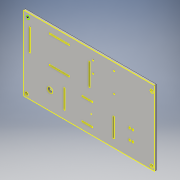
# Autodesk Inventor part: bottom
Saved by Autodesk Inventor 2016 (Build 200138000, 138)
## iProperties
Created: 2017-09-18
Part Number: bottom
Material: Generic
Document SubType Name: Modeling
Designer: Student
Density: 1 g/cm^3
Appearance: Default
Author: Student
Autodesk Inventor part; units mm, degrees
ref_plane "YZ Plane" through (0, 0, 0) normal (1, 0, 0) x (0, 1, 0)
ref_plane "XZ Plane" through (0, 0, 0) normal (0, 1, 0) x (-1, 0, 0)
ref_plane "XY Plane" through (0, 0, 0) normal (0, 0, 1) x (1, 0, 0)
sketch "Sketch1" plane through (0, 0, 0) normal (0, 0, 1) x (1, 0, 0)
  line L0 (-164.322, 128.7031) -> (152.924, 128.7031)
  line L1 (152.924, 128.7031) -> (152.924, -133.4523)
  line L2 (152.924, -133.4523) -> (-164.322, -133.4523)
  line L3 (-164.322, -133.4523) -> (-164.322, 128.7031)
  point P0 (0, 0)
  dimension "d0" = 317.246
  constraints: 8 end point, 2 parallel, 1 horizontal, 1 perpendicular
  measures "d0" distance of L0.start L0.end
extrude "Extrusion1" add sketch "Sketch1" along normal blind 4.699
sketch "Sketch2" plane through (0, 0, 4.699) normal (0, 0, 1) x (1, 0, 0)
  line L0 (-22.7697, 25.1619) -> (2.6303, 25.1619)
  line L1 (52.3147, 22.4498) -> (52.3147, -24.5402)
  line L2 (-64.5253, -24.5402) -> (-64.5253, 22.4498)
  line L3 (52.3147, 22.4498) -> (54.8547, 22.4498)
  line L4 (54.8547, 22.4498) -> (54.8547, -24.5402)
  line L5 (54.8547, -24.5402) -> (52.3147, -24.5402)
  line L6 (52.3147, -24.5402) -> (52.3147, 22.4498)
  line L7 (-64.5253, -24.5402) -> (-67.0653, -24.5402)
  line L8 (-67.0653, -24.5402) -> (-67.0653, 22.4498)
  line L9 (-67.0653, 22.4498) -> (-64.5253, 22.4498)
  line L10 (-64.5253, 22.4498) -> (-64.5253, -24.5402)
  line L11 (-22.7697, 25.1619) -> (2.6303, 25.1619)
  line L12 (2.6303, 25.1619) -> (2.6303, 27.7019)
  line L13 (2.6303, 27.7019) -> (-22.7697, 27.7019)
  line L14 (-22.7697, 27.7019) -> (-22.7697, 25.1619)
  line L15 (-22.7697, -25.2309) -> (2.6303, -25.2309)
  line L16 (2.6303, -25.2309) -> (2.6303, -27.7709)
  line L17 (2.6303, -27.7709) -> (-22.7697, -27.7709)
  line L18 (-22.7697, -27.7709) -> (-22.7697, -25.2309)
  circle A0 centre (92.5652, 17.0242) radius 2.286
  circle A1 centre (100.1852, 17.0242) radius 2.286
  circle A2 centre (92.5652, -8.3758) radius 2.286
  circle A3 centre (100.1852, -8.3758) radius 2.286
  line L19 (3.9163, 100.2262) -> (59.1645, 100.2262)
  circle A4 centre (54.7163, 69.5732) radius 1.397
  circle A5 centre (54.7163, 117.8332) radius 1.397
  circle A6 centre (3.9163, 114.6403) radius 1.397
  circle A7 centre (3.9163, 86.7003) radius 1.397
  point P0 (0, 0)
  dimension "d3" = 116.84
  dimension "d4" = 46.99
  dimension "d5" = 2.54
  dimension "d6" = 2.54
  dimension "d7" = 25.4
  dimension "d8" = 2.54
  dimension "d9" = 2.54
  dimension "d12" = 4.572
  dimension "d31" = 25.4
  dimension "d32" = 25.4
  constraints: 40 end point, 9 parallel, 8 centre point, 6 horizontal, 5 perpendicular, 1 point on line
  measures "d3" distance of L2.end L1.start
  measures "d4" distance of L1.start L1.end
  measures "d5" distance of L4.end L5.end
  measures "d6" distance of L8.end L9.end
  measures "d7" distance of L13.end L12.end
  measures "d8" distance of L0.end L12.end
  measures "d9" distance of L15.end L16.end
  measures "d12" diameter of A0
  measures "d31" distance of A3.centre A1.centre
  measures "d32" distance of A2.centre A0.centre
extrude "Extrusion2" cut sketch "Sketch2" against normal blind 25.4
sketch "Sketch3" plane through (0, 0, 4.699) normal (0, 0, 1) x (1, 0, 0)
  line L0 (-164.322, 128.7031) -> (-164.322, -133.4523) projected
  line L1 (152.924, 128.7031) -> (152.924, -133.4523) projected
  line L2 (-164.322, -44.2248) -> (152.924, -44.2248)
  line L3 (152.924, -44.2248) -> (152.924, -133.4523)
  line L4 (152.924, -133.4523) -> (-164.322, -133.4523)
  line L5 (-164.322, -133.4523) -> (-164.322, -44.2248)
  point P0 (0, 0)
  constraints: 8 end point, 2 parallel, 1 horizontal, 1 perpendicular, 1 point on line
extrude "Extrusion3" cut sketch "Sketch3" against normal blind 25.4
sketch "Sketch4" plane through (0, 0, 4.699) normal (0, 0, 1) x (1, 0, 0)
  line L0 (-102.2349, 116.84) -> (-53.5128, 116.84)
  line L1 (-6.2523, 108.1454) -> (-6.2523, 44.8408)
  line L2 (-53.5128, 53.5354) -> (-102.2349, 53.5354)
  line L3 (-148.4923, 53.5354) -> (-148.4923, 108.1454)
  line L4 (-148.4923, 108.1454) -> (-151.0323, 108.1454)
  line L5 (-151.0323, 108.1454) -> (-151.0323, 53.5354)
  line L6 (-151.0323, 53.5354) -> (-148.4923, 53.5354)
  line L7 (-148.4923, 53.5354) -> (-148.4923, 108.1454)
  line L8 (-6.2523, 108.1454) -> (-3.7123, 108.1454)
  line L9 (-3.7123, 108.1454) -> (-3.7123, 53.5354)
  line L10 (-3.7123, 53.5354) -> (-6.2523, 53.5354)
  line L11 (-6.2523, 53.5354) -> (-6.2523, 108.1454)
  line L12 (-102.2349, 116.84) -> (-53.5128, 116.84)
  line L13 (-53.5128, 116.84) -> (-53.5128, 119.5161)
  line L14 (-53.5128, 119.5161) -> (-102.2349, 119.5161)
  line L15 (-102.2349, 119.5161) -> (-102.2349, 116.84)
  line L16 (-102.2349, 53.5354) -> (-53.5128, 53.5354)
  line L17 (-53.5128, 53.5354) -> (-53.5128, 50.5868)
  line L18 (-53.5128, 50.5868) -> (-102.2349, 50.5868)
  line L19 (-102.2349, 50.5868) -> (-102.2349, 53.5354)
  circle A0 centre (-100.2931, 0) radius 6.35
  point P0 (0, 0)
  dimension "d21" = 142.24
  dimension "d22" = 2.54
  dimension "d23" = 2.54
  dimension "d24" = 12.7
  dimension "d25" = 54.61
  constraints: 40 end point, 10 parallel, 5 horizontal, 5 perpendicular, 3 point on line, 1 centre point
  measures "d21" distance of L3.end L1.start
  measures "d22" distance of L6.end L5.end
  measures "d23" distance of L9.end L10.end
  measures "d24" diameter of A0
  measures "d25" distance of L4.end L5.end
extrude "Extrusion4" cut sketch "Sketch4" against normal blind 25.4
sketch "Sketch5" plane through (0, 0, 4.699) normal (0, 0, 1) x (1, 0, 0)
  circle A0 centre (-154.2096, 125.6742) radius 4.064
  line L0 (-6.2523, 53.5354) -> (-6.2523, 108.1454) projected
  line L1 (-6.2523, 108.1454) -> (-3.7123, 108.1454) projected
  line L2 (-3.7123, 108.1454) -> (-3.7123, 53.5354) projected
  line L3 (-3.7123, 53.5354) -> (-6.2523, 53.5354) projected
  line L4 (-102.2349, 116.84) -> (-102.2349, 119.5161) projected
  line L5 (-102.2349, 119.5161) -> (-53.5128, 119.5161) projected
  line L6 (-53.5128, 119.5161) -> (-53.5128, 116.84) projected
  line L7 (-53.5128, 116.84) -> (-102.2349, 116.84) projected
  circle A1 centre (-100.2931, 0) radius 6.35 projected
  line L8 (-151.0323, 53.5354) -> (-151.0323, 108.1454) projected
  line L9 (-151.0323, 108.1454) -> (-148.4923, 108.1454) projected
  line L10 (-148.4923, 108.1454) -> (-148.4923, 53.5354) projected
  line L11 (-148.4923, 53.5354) -> (-151.0323, 53.5354) projected
  line L12 (-102.2349, 53.5354) -> (-53.5128, 53.5354) projected
  line L13 (-53.5128, 53.5354) -> (-53.5128, 50.5868) projected
  line L14 (-53.5128, 50.5868) -> (-102.2349, 50.5868) projected
  line L15 (-102.2349, 50.5868) -> (-102.2349, 53.5354) projected
  line L16 (-164.322, -44.2248) -> (152.924, -44.2248) projected
  line L17 (152.924, -44.2248) -> (152.924, 128.7031) projected
  line L18 (152.924, 128.7031) -> (-164.322, 128.7031) projected
  line L19 (-164.322, 128.7031) -> (-164.322, -44.2248) projected
  line L20 (-164.322, 128.7031) -> (152.924, 128.7031) projected
  line L21 (-5.699, 128.7031) -> (-5.699, 116.84)
  circle A2 centre (145.9955, 120.8351) radius 4.064
  line L22 (-164.322, -44.2248) -> (-164.322, 128.7031) projected
  line L23 (-164.322, 42.2392) -> (-157.3936, 42.2392)
  circle A3 centre (-157.3936, -36.3568) radius 4.064
  circle A4 centre (145.9955, -36.3568) radius 4.064
  point P0 (0, 0)
  dimension "d28" = 8.128
  constraints: 4 centre point, 4 end point, 2 midpoint, 1 horizontal, 1 symmetric about line, 1 vertical, 1 other
  measures "d28" diameter of A0
extrude "Extrusion5" cut sketch "Sketch5" against normal blind 25.4 contours A0 L18 | L18 A0 | A2 | A3 | A4
sketch "Sketch6" plane through (0, 0, 4.699) normal (0, 0, 1) x (1, 0, 0)
  circle A0 centre (-157.3936, -36.3568) radius 4.064 projected
  arc A1 (-156.9191, 128.7031) -> (-151.5, 128.7031) centre (-154.2096, 125.6742) ccw projected
  circle A2 centre (145.9955, 120.8351) radius 4.064 projected
  circle A3 centre (145.9955, -36.3568) radius 4.064 projected
  line L0 (-6.2523, 53.5354) -> (-6.2523, 108.1454) projected
  line L1 (-6.2523, 108.1454) -> (-3.7123, 108.1454) projected
  line L2 (-3.7123, 108.1454) -> (-3.7123, 53.5354) projected
  line L3 (-3.7123, 53.5354) -> (-6.2523, 53.5354) projected
  line L4 (-102.2349, 116.84) -> (-102.2349, 119.5161) projected
  line L5 (-102.2349, 119.5161) -> (-53.5128, 119.5161) projected
  line L6 (-53.5128, 119.5161) -> (-53.5128, 116.84) projected
  line L7 (-53.5128, 116.84) -> (-102.2349, 116.84) projected
  circle A4 centre (-100.2931, 0) radius 6.35 projected
  line L8 (-151.0323, 53.5354) -> (-151.0323, 108.1454) projected
  line L9 (-151.0323, 108.1454) -> (-148.4923, 108.1454) projected
  line L10 (-148.4923, 108.1454) -> (-148.4923, 53.5354) projected
  line L11 (-148.4923, 53.5354) -> (-151.0323, 53.5354) projected
  line L12 (-102.2349, 53.5354) -> (-53.5128, 53.5354) projected
  line L13 (-53.5128, 53.5354) -> (-53.5128, 50.5868) projected
  line L14 (-53.5128, 50.5868) -> (-102.2349, 50.5868) projected
  line L15 (-102.2349, 50.5868) -> (-102.2349, 53.5354) projected
  line L16 (-164.322, -44.2248) -> (152.924, -44.2248) projected
  line L17 (152.924, -44.2248) -> (152.924, 128.7031) projected
  line L18 (152.924, 128.7031) -> (-151.5, 128.7031) projected
  line L19 (-164.322, 128.7031) -> (-164.322, -44.2248) projected
  line L20 (-64.5253, 22.4498) -> (-64.5253, -24.5402) projected
  line L21 (-64.5253, -24.5402) -> (-67.0653, -24.5402) projected
  line L22 (-67.0653, -24.5402) -> (-67.0653, 22.4498) projected
  line L23 (-67.0653, 22.4498) -> (-64.5253, 22.4498) projected
  line L24 (-22.7697, -27.7709) -> (-22.7697, -25.2309) projected
  line L25 (-22.7697, -25.2309) -> (2.6303, -25.2309) projected
  line L26 (2.6303, -25.2309) -> (2.6303, -27.7709) projected
  line L27 (2.6303, -27.7709) -> (-22.7697, -27.7709) projected
  circle A5 centre (100.1852, -8.3758) radius 2.286 projected
  circle A6 centre (100.1852, 17.0242) radius 2.286 projected
  circle A7 centre (54.7163, 117.8332) radius 1.397 projected
  circle A8 centre (54.7163, 69.5732) radius 1.397 projected
  circle A9 centre (3.9163, 86.7003) radius 1.397 projected
  circle A10 centre (3.9163, 114.6403) radius 1.397 projected
  circle A11 centre (92.5652, 17.0242) radius 2.286 projected
  circle A12 centre (92.5652, -8.3758) radius 2.286 projected
  line L28 (-22.7697, 25.1619) -> (-22.7697, 27.7019) projected
  line L29 (-22.7697, 27.7019) -> (2.6303, 27.7019) projected
  line L30 (2.6303, 27.7019) -> (2.6303, 25.1619) projected
  line L31 (2.6303, 25.1619) -> (-22.7697, 25.1619) projected
  line L32 (52.3147, -24.5402) -> (52.3147, 22.4498) projected
  line L33 (52.3147, 22.4498) -> (54.8547, 22.4498) projected
  line L34 (54.8547, 22.4498) -> (54.8547, -24.5402) projected
  line L35 (54.8547, -24.5402) -> (52.3147, -24.5402) projected
  line L36 (-164.322, 128.7031) -> (152.924, 128.7031) projected
  line L37 (-164.322, 128.7031) -> (152.924, 128.7031)
  line L38 (152.924, 128.7031) -> (152.924, 136.3029)
  line L39 (152.924, 136.3029) -> (-164.322, 136.3029)
  line L40 (-164.322, 136.3029) -> (-164.322, 128.7031)
  line L41 (-156.9191, 128.7031) -> (-164.322, 128.7031) projected
  point P0 (0, 0)
  constraints: 8 end point, 2 parallel, 1 horizontal, 1 perpendicular
extrude "Extrusion6" add sketch "Sketch6" against normal blind 4.699 contours L36 L40 L39 L38 L18
sketch "Sketch7" plane through (0, 0, 4.699) normal (0, 0, 1) x (1, 0, 0)
  arc A0 (-156.9191, 128.7031) -> (-151.5, 128.7031) centre (-154.2096, 125.6742) ccw projected
  line L0 (-156.9191, 128.7031) -> (-151.5, 128.7031) projected
  line L1 (152.924, -44.2248) -> (152.924, 136.3029) projected
  line L2 (152.924, 136.3029) -> (-164.322, 136.3029) projected
  line L3 (-164.322, 136.3029) -> (-164.322, -44.2248) projected
  line L4 (-164.322, -44.2248) -> (152.924, -44.2248) projected
  circle A1 centre (-157.3936, -36.3568) radius 4.064 projected
  circle A2 centre (145.9955, 120.8351) radius 4.064 projected
  circle A3 centre (145.9955, -36.3568) radius 4.064 projected
  line L5 (-6.2523, 53.5354) -> (-6.2523, 108.1454) projected
  line L6 (-6.2523, 108.1454) -> (-3.7123, 108.1454) projected
  line L7 (-3.7123, 108.1454) -> (-3.7123, 53.5354) projected
  line L8 (-3.7123, 53.5354) -> (-6.2523, 53.5354) projected
  line L9 (-102.2349, 116.84) -> (-102.2349, 119.5161) projected
  line L10 (-102.2349, 119.5161) -> (-53.5128, 119.5161) projected
  line L11 (-53.5128, 119.5161) -> (-53.5128, 116.84) projected
  line L12 (-53.5128, 116.84) -> (-102.2349, 116.84) projected
  circle A4 centre (-100.2931, 0) radius 6.35 projected
  line L13 (-151.0323, 53.5354) -> (-151.0323, 108.1454) projected
  line L14 (-151.0323, 108.1454) -> (-148.4923, 108.1454) projected
  line L15 (-148.4923, 108.1454) -> (-148.4923, 53.5354) projected
  line L16 (-148.4923, 53.5354) -> (-151.0323, 53.5354) projected
  line L17 (-102.2349, 53.5354) -> (-53.5128, 53.5354) projected
  line L18 (-53.5128, 53.5354) -> (-53.5128, 50.5868) projected
  line L19 (-53.5128, 50.5868) -> (-102.2349, 50.5868) projected
  line L20 (-102.2349, 50.5868) -> (-102.2349, 53.5354) projected
  line L21 (-64.5253, 22.4498) -> (-64.5253, -24.5402) projected
  line L22 (-64.5253, -24.5402) -> (-67.0653, -24.5402) projected
  line L23 (-67.0653, -24.5402) -> (-67.0653, 22.4498) projected
  line L24 (-67.0653, 22.4498) -> (-64.5253, 22.4498) projected
  line L25 (-22.7697, -27.7709) -> (-22.7697, -25.2309) projected
  line L26 (-22.7697, -25.2309) -> (2.6303, -25.2309) projected
  line L27 (2.6303, -25.2309) -> (2.6303, -27.7709) projected
  line L28 (2.6303, -27.7709) -> (-22.7697, -27.7709) projected
  circle A5 centre (100.1852, -8.3758) radius 2.286 projected
  circle A6 centre (100.1852, 17.0242) radius 2.286 projected
  circle A7 centre (54.7163, 117.8332) radius 1.397 projected
  circle A8 centre (54.7163, 69.5732) radius 1.397 projected
  circle A9 centre (3.9163, 86.7003) radius 1.397 projected
  circle A10 centre (3.9163, 114.6403) radius 1.397 projected
  circle A11 centre (92.5652, 17.0242) radius 2.286 projected
  circle A12 centre (92.5652, -8.3758) radius 2.286 projected
  line L29 (-22.7697, 25.1619) -> (-22.7697, 27.7019) projected
  line L30 (-22.7697, 27.7019) -> (2.6303, 27.7019) projected
  line L31 (2.6303, 27.7019) -> (2.6303, 25.1619) projected
  line L32 (2.6303, 25.1619) -> (-22.7697, 25.1619) projected
  line L33 (52.3147, -24.5402) -> (52.3147, 22.4498) projected
  line L34 (52.3147, 22.4498) -> (54.8547, 22.4498) projected
  line L35 (54.8547, 22.4498) -> (54.8547, -24.5402) projected
  line L36 (54.8547, -24.5402) -> (52.3147, -24.5402) projected
  circle A13 centre (-154.2096, 125.6742) radius 4.064
  point P0 (0, 0)
  constraints: 1 centre point, 1 coincident
body "Solid1"
